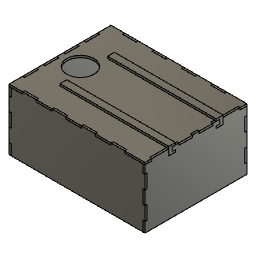
prototype v2 (Autodesk Fusion 360 design; units mm, degrees)
Autodesk Fusion 360 part; units mm, degrees
note: some values were not read from the file. Set by a fixed rule: which sketch regions a step uses.
sketch "Sketch1" plane through (0, 0, 0) normal (0, 1, 0) x (1, 0, 0)
  line L0 (0, 0) -> (200, 0)
  line L1 (200, 0) -> (200, -150)
  line L2 (200, -150) -> (0, -150)
  line L3 (0, -150) -> (0, 0)
  line L4 (0, -20) -> (3, -20)
  line L5 (3, -20) -> (3, -40)
  line L6 (3, -40) -> (0, -40)
  line L7 (0, -40) -> (0, -20)
  line L8 (3, -70) -> (0, -70)
  line L9 (3, -50) -> (3, -70)
  line L10 (0, -50) -> (3, -50)
  line L11 (3, -100) -> (0, -100)
  line L12 (3, -80) -> (3, -100)
  line L13 (0, -80) -> (3, -80)
  line L14 (3, -130) -> (0, -130)
  line L15 (3, -110) -> (3, -130)
  line L16 (0, -110) -> (3, -110)
  line L17 (170, 0) -> (150, 0)
  line L18 (150, 0) -> (150, -3)
  line L19 (150, -3) -> (170, -3)
  line L20 (170, -3) -> (170, 0)
  line L21 (170, -150) -> (150, -150)
  line L22 (150, -150) -> (150, -147)
  line L23 (150, -147) -> (170, -147)
  line L24 (170, -147) -> (170, -150)
  line L25 (-40, -147) -> (-40, -150)
  line L26 (200, -40) -> (200, -35)
  line L27 (200, -110) -> (40, -110)
  line L28 (40, -110) -> (40, -115)
  line L29 (40, -115) -> (200, -115)
  line L30 (200, -115) -> (200, -110)
  line L31 (200, -120) -> (200, -140)
  line L32 (200, -10.0504) -> (197, -10.0504)
  line L33 (197, -10.0504) -> (197, -30.0504)
  line L34 (197, -30.0504) -> (200, -30.0504)
  line L35 (200, -30.0504) -> (200, -10.0504)
  line L36 (200, -50) -> (197, -50)
  line L37 (197, -50) -> (197, -70)
  line L38 (197, -70) -> (200, -70)
  line L39 (200, -70) -> (200, -50)
  line L40 (200, -80) -> (197, -80)
  line L41 (197, -80) -> (197, -100)
  line L42 (197, -100) -> (200, -100)
  line L43 (30, 0) -> (30, -150) construction
  line L44 (0, -75) -> (30, -75) construction
  circle A0 centre (30, -75) radius 20
  line L45 (46.6667, -115) -> (53.3333, -110) construction
  line L46 (200, -35) -> (40, -35)
  line L47 (40, -35) -> (40, -40)
  line L48 (40, -40) -> (200, -40)
  line L49 (200, -40) -> (200, -35)
  line L50 (106.6667, -3) -> (126.6667, -3)
  line L51 (106.6667, 0) -> (106.6667, -3)
  line L52 (126.6667, -3) -> (126.6667, 0)
  line L53 (63.3333, -3) -> (83.3333, -3)
  line L54 (63.3333, 0) -> (63.3333, -3)
  line L55 (83.3333, -3) -> (83.3333, 0)
  line L56 (20, -3) -> (40, -3)
  line L57 (20, 0) -> (20, -3)
  line L58 (40, -3) -> (40, 0)
  line L59 (106.6667, -147) -> (126.6667, -147)
  line L60 (126.6667, -147) -> (126.6667, -150)
  line L61 (106.6667, -150) -> (106.6667, -147)
  line L62 (63.3333, -147) -> (83.3333, -147)
  line L63 (83.3333, -147) -> (83.3333, -150)
  line L64 (63.3333, -150) -> (63.3333, -147)
  line L65 (20, -147) -> (40, -147)
  line L66 (40, -147) -> (40, -150)
  line L67 (20, -150) -> (20, -147)
  line L68 (200, -120) -> (197, -120)
  line L69 (197, -120) -> (197, -140)
  line L70 (197, -140) -> (200, -140)
  line L71 (200, -140) -> (200, -120)
  line L72 (197, -150) -> (197, 0)
  point P0 (0, -20)
  point P1 (170, 0)
  point P2 (170, -150)
  point P3 (200, -35)
  point P4 (200, -110)
  point P5 (30, 0)
  point P6 (197, -150)
  dimension "d1" = 200
  dimension "d2" = 150
  dimension "d10" = 20
  dimension "d11" = 3
  dimension "d12" = 20
  dimension "d15" = 0
  dimension "d16" = -90
  dimension "d17" = 30
  dimension "d18" = 20
  dimension "d19" = 3
  dimension "d24" = 30
  dimension "d25" = 20
  dimension "d31" = 35
  dimension "d37" = 70
  dimension "d39" = 5
  dimension "d44" = 3
  dimension "d48" = 0
  dimension "d49" = -30
  dimension "d155" = 30
  dimension "d157" = 40
  dimension "d158" = 160
  dimension "d162" = -130
  dimension "d163" = 0
  dimension "d166" = -130
  dimension "d167" = 0
  constraint horizontal L0
  constraint vertical L1
  constraint horizontal L2
  constraint vertical L3
  constraint coincident L0.start L3.end
  constraint coincident L3 P0
  constraint horizontal L4
  constraint vertical L5
  constraint horizontal L6
  constraint vertical L7
  constraint coincident P0 L4.start
  constraint coincident L0 P1
  constraint horizontal L17
  constraint vertical L18
  constraint horizontal L19
  constraint vertical L20
  constraint coincident P1 L17.start
  constraint coincident L2 P2
  constraint horizontal L21
  constraint vertical L22
  constraint horizontal L23
  constraint vertical L24
  constraint coincident P2 L21.start
  constraint coincident L1 P3
  constraint vertical L26
  constraint coincident P3 L26.end
  constraint coincident L1 P4
  constraint horizontal L27
  constraint vertical L28
  constraint horizontal L29
  constraint vertical L30
  constraint coincident P4 L27.start
  constraint vertical L31
  constraint coincident L1 L31.end
  constraint horizontal L32
  constraint vertical L33
  constraint horizontal L34
  constraint vertical L35
  constraint coincident L1 L32.start
  constraint horizontal L36
  constraint vertical L37
  constraint horizontal L38
  constraint vertical L39
  constraint coincident L1 L36.start
  constraint coincident L0 P5
  constraint coincident P5 L43.start
  constraint coincident L2 L43.end
  constraint perpendicular L2 L43
  constraint midpoint L3 L44.start
  constraint midpoint L43 L44.end
  constraint coincident L44.end A0.centre
  constraint coincident L27 L45.end
  constraint coincident L29 L45.start
  constraint horizontal L46
  constraint vertical L47
  constraint horizontal L48
  constraint vertical L49
  constraint horizontal L68
  constraint vertical L69
  constraint horizontal L70
  constraint vertical L71
  constraint coincident L2 P6
  constraint coincident P6 L72.start
  measures "d1" distance of L0.start L0.end
  measures "d2" distance of L0.start L2.end
  measures "d10" distance of L0.start L4.start
  measures "d11" distance of P0 L4.end
  measures "d12" distance of P0 L6.end
  measures "d17" distance of L1 P1
  measures "d18" distance of P1 L17.end
  measures "d19" distance of P1 L19.end
  measures "d24" distance of L1.end P2
  measures "d25" distance of P2 L21.end
  measures "d31" distance of L0.end P3
  measures "d37" distance of L26.start P4
  measures "d39" distance of P4 L29.end
  measures "d44" distance of L36.start L36.end
  measures "d155" distance of L0.start P5
  measures "d157" diameter of A0
  measures "d158" distance of P3 L46.end
extrude "Extrude1" add sketch "Sketch1" against normal blind 3 contours L0 L2 L3 L4 L5 L6 L8 L9 L10 L11 L12 L13 L14 L15 L16 L18 L19 L20 L22 L23 L24 L27 L28 L29 L33 L37 L41 L46 L47 L48 L50 L51 L52 L53 L54 L55 L56 L57 L58 L59 L60 L61 L62 L63 L64 L65 L66 L67 L69 L72 | L0 L1 L32 L72 | L1 L36 L37 L38 L39 L72 | L1 L40 L41 L42 L72 | L1 L2 L70 L72 makes body 1
sketch "Sketch2" plane through (0, 0, 150) normal (0, 0, 1) x (1, 0, 0)
  line L0 (200, 0) -> (200, -90)
  line L1 (200, -90) -> (0, -90)
  line L2 (0, -90) -> (0, 0)
  line L3 (0, -3) -> (0, 0)
  line L4 (200, -3) -> (200, 0)
  line L5 (0, -35) -> (0, -15)
  line L6 (0, -15) -> (3, -15)
  line L7 (3, -15) -> (3, -35)
  line L8 (3, -35) -> (0, -35)
  line L9 (0, -35) -> (0, -15)
  line L10 (0, -55) -> (3, -55)
  line L11 (3, -55) -> (3, -75)
  line L12 (3, -75) -> (0, -75)
  line L13 (3, -35) -> (3, -55)
  line L14 (3, -75) -> (3, -90)
  line L15 (200, -15) -> (197, -15)
  line L16 (197, -15) -> (197, -35)
  line L17 (197, -35) -> (200, -35)
  line L18 (200, -35) -> (200, -15)
  line L19 (200, -55) -> (197, -55)
  line L20 (197, -55) -> (197, -75)
  line L21 (197, -75) -> (200, -75)
  line L22 (0, 0) -> (200, 0)
  line L23 (3, -15) -> (3, 0)
  line L24 (170, 0) -> (150, 0)
  line L25 (150, 0) -> (150, -3)
  line L26 (150, -3) -> (170, -3)
  line L27 (170, -3) -> (170, 0)
  line L28 (106.6667, -3) -> (126.6667, -3)
  line L29 (106.6667, 0) -> (106.6667, -3)
  line L30 (126.6667, -3) -> (126.6667, 0)
  line L31 (63.3333, -3) -> (83.3333, -3)
  line L32 (63.3333, 0) -> (63.3333, -3)
  line L33 (83.3333, -3) -> (83.3333, 0)
  line L34 (20, -3) -> (40, -3)
  line L35 (20, 0) -> (20, -3)
  line L36 (40, -3) -> (40, 0)
  line L37 (200, -3) -> (0, -3)
  line L38 (197, -3) -> (197, -90)
  point P0 (0, -15)
  point P1 (0, -55)
  point P2 (200, -15)
  point P3 (0, -3)
  point P4 (200, -3)
  point P5 (170, 0)
  point P6 (197, -3)
  dimension "d61" = 200
  dimension "d62" = 90
  dimension "d98" = 15
  dimension "d105" = 0
  dimension "d106" = -40
  dimension "d116" = 20
  dimension "d119" = 0
  dimension "d120" = -40
  dimension "d180" = -130
  dimension "d181" = 0
  constraint vertical L0
  constraint vertical L2
  constraint coincident L2.end L3.end
  constraint vertical L3
  constraint vertical L4
  constraint coincident L2 P0
  constraint vertical L5
  constraint coincident P0 L5.end
  constraint horizontal L6
  constraint vertical L7
  constraint horizontal L8
  constraint vertical L9
  constraint coincident L2 P1
  constraint coincident L1 L14.end
  constraint coincident L0 P2
  constraint horizontal L15
  constraint vertical L16
  constraint horizontal L17
  constraint vertical L18
  constraint coincident P2 L15.start
  constraint perpendicular L0 L22
  constraint coincident L22 L23.end
  constraint perpendicular L22 L23
  constraint horizontal L24
  constraint vertical L25
  constraint horizontal L26
  constraint vertical L27
  constraint coincident P5 L24.start
  constraint coincident P4 L4.start
  constraint perpendicular L0 L37
  constraint coincident L37 P6
  constraint coincident P6 L38.start
  constraint coincident L1 L38.end
  constraint perpendicular L1 L38
  measures "d61" distance of L2.end L0.start
  measures "d62" distance of L2.end L1.end
  measures "d98" distance of L2.end L5.end
  measures "d116" distance of P2 L17.end
extrude "Extrude4" add sketch "Sketch2" against normal blind 3 separate body contours L22 L24 L25 L26 L27 L37 | L0 L15 L16 L17 L18 L38 | L1 L7 L11 L13 L14 L16 L20 L23 L26 L28 L31 L34 L37 L38 | L22 L28 L29 L30 L37 | L0 L19 L20 L21 L38 | L22 L31 L32 L33 L37 | L22 L34 L35 L36 L37 | L2 L10 L11 L12 | L2 L5 L6 L7 L8 L9 makes body 2
sketch "Sketch3" plane through (0, 0, 0) normal (0, 0, -1) x (-1, 0, 0)
  line L0 (-200, 0) -> (-200, -90)
  line L1 (-200, -90) -> (0, -90)
  line L2 (0, -90) -> (0, 0)
  line L3 (-200, -3) -> (-200, 0)
  line L4 (0, -3) -> (0, 0)
  line L5 (-3, -15) -> (-3, 0)
  line L6 (-3, -15) -> (-3, -90)
  line L7 (-3, -15) -> (0, -15)
  line L8 (-3, -35) -> (0, -35)
  line L9 (-3, -55) -> (0, -55)
  line L10 (0, -75) -> (-3, -75)
  line L11 (-200, -15) -> (-197, -15)
  line L12 (-197, -15) -> (-197, -35)
  line L13 (-197, -35) -> (-200, -35)
  line L14 (-200, -35) -> (-200, -15)
  line L15 (-170, 0) -> (-150, 0)
  line L16 (-150, 0) -> (-150, -3)
  line L17 (-150, -3) -> (-170, -3)
  line L18 (-170, -3) -> (-170, 0)
  line L19 (-126.6667, -3) -> (-126.6667, 0)
  line L20 (-106.6667, -3) -> (-126.6667, -3)
  line L21 (-106.6667, 0) -> (-106.6667, -3)
  line L22 (-83.3333, -3) -> (-83.3333, 0)
  line L23 (-63.3333, -3) -> (-83.3333, -3)
  line L24 (-63.3333, 0) -> (-63.3333, -3)
  line L25 (-40, -3) -> (-40, 0)
  line L26 (-20, -3) -> (-40, -3)
  line L27 (-20, 0) -> (-20, -3)
  line L28 (-200, -90) -> (-3, -90)
  line L29 (-200, 0) -> (0, 0)
  line L30 (0, -3) -> (-200, -3)
  line L31 (-200, -55) -> (-197, -55)
  line L32 (-197, -55) -> (-197, -75)
  line L33 (-197, -75) -> (-200, -75)
  line L34 (-200, -75) -> (-200, -55)
  line L35 (-197, -90) -> (-197, 0)
  point P0 (-3, -35)
  point P1 (-3, -55)
  point P2 (-3, -75)
  point P3 (-200, -15)
  point P4 (0, -3)
  point P5 (-170, 0)
  point P6 (-150, -3)
  point P7 (-3, -15)
  point P8 (0, -15)
  point P9 (-200, -55)
  point P10 (-197, -90)
  dimension "d65" = 200
  dimension "d66" = 90
  dimension "d108" = 3
  dimension "d172" = 130
  dimension "d173" = 0
  constraint vertical L0
  constraint coincident L2.end L4.end
  constraint coincident L2 P8
  constraint coincident P0 L8.start
  constraint coincident L2 L8.end
  constraint coincident P1 L9.start
  constraint coincident L2 L9.end
  constraint coincident L2 L10.start
  constraint coincident P2 L10.end
  constraint perpendicular L6 L10
  constraint coincident L0 P3
  constraint horizontal L11
  constraint vertical L12
  constraint horizontal L13
  constraint vertical L14
  constraint coincident P3 L11.start
  constraint horizontal L15
  constraint vertical L16
  constraint horizontal L17
  constraint vertical L18
  constraint coincident P6 L16.end
  constraint coincident P5 L15.start
  constraint perpendicular L2 L29
  constraint perpendicular L3 L30
  constraint horizontal L31
  constraint vertical L32
  constraint horizontal L33
  constraint vertical L34
  constraint coincident P9 L31.start
  constraint coincident P10 L35.start
  constraint coincident L29 L35.end
  measures "d65" distance of L2.end L0.start
  measures "d66" distance of L2.end L1.end
  measures "d108" distance of P3 L11.end
extrude "Extrude12" add sketch "Sketch3" against normal blind 3 separate body contours L0 L11 L12 L13 L14 L35 | L1 L5 L6 L12 L17 L20 L23 L26 L28 L30 L32 L35 | L15 L16 L17 L18 L29 L30 | L0 L31 L32 L33 L34 L35 | L19 L20 L21 L29 L30 | L22 L23 L24 L29 L30 | L25 L26 L27 L29 L30 | L2 L6 L9 L10 | L2 L6 L7 L8 makes body 3
sketch "Sketch4" plane through (200, 0, 0) normal (1, 0, 0) x (0, 0, -1)
  line L0 (-140, 0) -> (-150, 0)
  line L1 (-150, 0) -> (-150, -3)
  line L2 (-150, -3) -> (-140, -3)
  line L3 (0, 0) -> (-150, 0)
  line L4 (-150, 0) -> (-150, -90)
  line L5 (-150, -90) -> (0, -90)
  line L6 (0, -90) -> (0, 0)
  line L7 (-10.0504, -3) -> (0, -3)
  line L8 (0, -3) -> (0, 0)
  line L9 (0, 0) -> (-10.0504, 0)
  line L10 (-10.0504, 0) -> (-10.0504, -3)
  line L11 (-30.0504, -3) -> (-35, -3)
  line L12 (-35, -3) -> (-35, 0)
  line L13 (-35, 0) -> (-30.0504, 0)
  line L14 (-30.0504, 0) -> (-30.0504, -3)
  line L15 (-40, -3) -> (-50, -3)
  line L16 (-50, -3) -> (-50, 0)
  line L17 (-50, 0) -> (-40, 0)
  line L18 (-40, 0) -> (-40, -3)
  line L19 (-70, -3) -> (-80, -3)
  line L20 (-80, -3) -> (-80, 0)
  line L21 (-80, 0) -> (-70, 0)
  line L22 (-70, 0) -> (-70, -3)
  line L23 (-100, -3) -> (-110, -3)
  line L24 (-110, -3) -> (-110, 0)
  line L25 (-110, 0) -> (-100, 0)
  line L26 (-100, 0) -> (-100, -3)
  line L27 (-115, -3) -> (-120, -3)
  line L28 (-120, -3) -> (-120, 0)
  line L29 (-120, 0) -> (-115, 0)
  line L30 (-115, 0) -> (-115, -3)
  line L31 (-140, -3) -> (-150, -3)
  line L32 (-150, -3) -> (-150, 0)
  line L33 (-150, 0) -> (-140, 0)
  line L34 (-140, 0) -> (-140, -3)
  line L35 (-115, -3) -> (-110, -3)
  line L36 (-40, -3) -> (-35, -3)
  line L37 (-115, -3) -> (-110, -3)
  line L38 (-35, -3) -> (-45, -3)
  line L39 (-150, -15) -> (-147, -15)
  line L40 (-147, -15) -> (-147, -35)
  line L41 (-147, -35) -> (-150, -35)
  line L42 (-150, -35) -> (-150, -15)
  line L43 (-150, -55) -> (-147, -55)
  line L44 (-147, -55) -> (-147, -75)
  line L45 (-147, -75) -> (-150, -75)
  line L46 (-147, -15, 0) -> (-147, -90, -3)
  line L47 (-147, -15) -> (-147, 0)
  line L48 (0, -15) -> (-3, -15)
  line L49 (-3, -15) -> (-3, -35)
  line L50 (-3, -35) -> (0, -35)
  line L51 (0, -35) -> (0, -15)
  line L52 (0, -55) -> (-3, -55)
  line L53 (-3, -55) -> (-3, -75)
  line L54 (-3, -75) -> (0, -75)
  line L55 (-3.0756, 0) -> (-3.0756, -90)
  line L56 (-115, -3) -> (-105, -3)
  line L57 (-105, -9) -> (-115, -9)
  line L58 (-115, -9) -> (-115, -3)
  line L59 (-35, -3) -> (-45, -3)
  line L60 (-45, -9) -> (-35, -9)
  line L61 (-35, -9) -> (-35, -3)
  line L62 (-110, -3) -> (-110, -6)
  line L63 (-110, -6) -> (-105, -6)
  line L64 (-105, -6) -> (-105, -9)
  line L65 (-40, -3) -> (-40, -6)
  line L66 (-40, -6) -> (-45, -6)
  line L67 (-45, -6) -> (-45, -9)
  line L68 (-115, 0) -> (-104.994, 0)
  line L69 (-104.994, 0) -> (-104.994, 3)
  line L70 (-104.994, 3) -> (-115, 3)
  line L71 (-115, 3) -> (-115, 0)
  line L72 (-35, 0) -> (-45, 0)
  line L73 (-45, 0) -> (-45, 3)
  line L74 (-45, 3) -> (-35, 3)
  line L75 (-35, 3) -> (-35, 0)
  line L76 (-140, -3) -> (-140, 0)
  line L77 (-150, -3) -> (0, -3)
  point P0 (-70, -3)
  point P1 (-30.0504, -3)
  point P2 (-10.0504, -3)
  point P3 (-150, -15)
  point P4 (0, -15)
  point P5 (-115, -3)
  point P6 (-115, 0)
  point P7 (-147, -90)
  point P8 (-30.0504, -3)
  point P9 (-30.0504, 0)
  point P10 (-150, -3)
  point P11 (-140, -3)
  point P12 (-120, -3)
  point P13 (-35, -3)
  point P14 (-35, 0)
  point P15 (-120, 0)
  point P16 (-115, -3)
  point P17 (-110, -3)
  point P18 (-100, -3)
  point P19 (-80, -3)
  point P20 (-50, -3)
  point P21 (-50, -3)
  point P22 (-70, -3)
  point P23 (-50, 0)
  point P24 (-80, 0)
  point P25 (-110, 0)
  point P26 (-110, 0)
  point P27 (-150, -15)
  point P28 (-147, -90)
  dimension "d69" = 150
  dimension "d70" = 90
  dimension "d79" = 10
  dimension "d122" = 3
  dimension "d123" = 20
  dimension "d126" = 0
  dimension "d127" = -40
  dimension "d129" = 3
  dimension "d130" = 20
  dimension "d133" = 0
  dimension "d134" = -40
  dimension "d143" = 10
  dimension "d144" = 6
  dimension "d145" = 10
  dimension "d146" = 6
  dimension "d147" = 3
  dimension "d153" = 3
  dimension "d154" = 3
  dimension "d185" = 150
  constraint horizontal L3
  constraint vertical L4
  constraint horizontal L5
  constraint vertical L6
  constraint coincident L3.start L6.end
  constraint horizontal L7
  constraint vertical L8
  constraint horizontal L9
  constraint vertical L10
  constraint coincident P2 L7.start
  constraint horizontal L11
  constraint vertical L12
  constraint horizontal L13
  constraint vertical L14
  constraint coincident P8 P1
  constraint horizontal L15
  constraint vertical L16
  constraint horizontal L17
  constraint vertical L18
  constraint horizontal L19
  constraint vertical L20
  constraint horizontal L21
  constraint vertical L22
  constraint coincident P22 P0
  constraint horizontal L23
  constraint vertical L24
  constraint horizontal L25
  constraint vertical L26
  constraint horizontal L27
  constraint vertical L28
  constraint horizontal L29
  constraint vertical L30
  constraint horizontal L31
  constraint vertical L32
  constraint horizontal L33
  constraint vertical L34
  constraint coincident L0.end L1.start
  constraint coincident P17 L23.end
  constraint horizontal L37
  constraint horizontal L38
  constraint horizontal L39
  constraint vertical L40
  constraint horizontal L41
  constraint vertical L42
  constraint coincident L3 L47.end
  constraint coincident L6 P4
  constraint horizontal L48
  constraint vertical L49
  constraint horizontal L50
  constraint vertical L51
  constraint coincident P4 L48.start
  constraint coincident L3 L55.start
  constraint coincident L5 L55.end
  constraint perpendicular L5 L55
  constraint horizontal L56
  constraint horizontal L57
  constraint vertical L58
  constraint horizontal L59
  constraint horizontal L60
  constraint vertical L61
  constraint perpendicular L56 L62
  constraint perpendicular L62 L63
  constraint perpendicular L38 L65
  constraint perpendicular L65 L66
  constraint horizontal L68
  constraint vertical L69
  constraint horizontal L70
  constraint vertical L71
  constraint horizontal L72
  constraint vertical L73
  constraint horizontal L74
  constraint vertical L75
  constraint perpendicular L4 L77
  measures "d69" distance of L3.start L0.end
  measures "d70" distance of L3.start L5.end
  measures "d79" distance of P13 L38.end
  measures "d122" distance of P27 L39.end
  measures "d123" distance of P27 L41.end
  measures "d129" distance of P4 L48.end
  measures "d130" distance of P4 L50.end
  measures "d143" distance of P16 L56.end
  measures "d144" distance of P16 L57.end
  measures "d145" distance of P13 L38.end
  measures "d146" distance of P13 L60.end
  measures "d147" distance of P17 L62.end
  measures "d153" distance of P6 L70.end
  measures "d154" distance of P14 L74.end
  measures "d185" distance of P10 L7.end
extrude "Extrude6" add sketch "Sketch4" against normal blind 3 separate body contours L3 L28 L34 L76 L77 | L3 L27 L28 L29 L30 L77 | L2 L4 L5 L7 L11 L15 L19 L23 L27 L31 L38 L40 L41 L43 L44 L45 L47 L55 L56 L57 L58 L59 L60 L61 L62 L63 L64 L65 L66 L67 L77 | L2 L4 L31 L39 L47 L77 | L3 L23 L24 L25 L26 L56 L68 L77 | L3 L19 L20 L21 L22 L77 | L3 L15 L16 L17 L18 L38 L59 L72 L77 | L5 L6 L7 L48 L49 L50 L52 L53 L54 L55 L77 | L3 L10 L14 L77 | L3 L11 L12 L13 L14 L77 makes body 4
sketch "Sketch5" plane through (0, 0, 0) normal (-1, 0, 0) x (0, 0, 1)
  line L0 (50, 0) -> (40, 0)
  line L1 (40, 0) -> (40, -3)
  line L2 (40, -3) -> (50, -3)
  line L3 (50, -3) -> (50, 0)
  line L4 (0, 0) -> (150, 0)
  line L5 (150, 0) -> (150, -90)
  line L6 (150, -90) -> (0, -90)
  line L7 (0, -90) -> (0, 0)
  line L8 (130, -3) -> (150, -3)
  line L9 (150, -3) -> (150, 0)
  line L10 (150, 0) -> (130, 0)
  line L11 (130, 0) -> (130, -3)
  line L12 (110, -3) -> (100, -3)
  line L13 (100, -3) -> (100, 0)
  line L14 (100, 0) -> (110, 0)
  line L15 (110, 0) -> (110, -3)
  line L16 (80, -3) -> (70, -3)
  line L17 (70, -3) -> (70, 0)
  line L18 (70, 0) -> (80, 0)
  line L19 (80, 0) -> (80, -3)
  line L20 (50, -3) -> (40, -3)
  line L21 (40, -3) -> (40, 0)
  line L22 (40, 0) -> (50, 0)
  line L23 (50, 0) -> (50, -3)
  line L24 (20, -3) -> (0, -3)
  line L25 (0, -3) -> (0, 0)
  line L26 (0, 0) -> (20, 0)
  line L27 (20, 0) -> (20, -3)
  line L28 (150, -15) -> (147, -15)
  line L29 (147, -15) -> (147, -35)
  line L30 (147, -35) -> (150, -35)
  line L31 (150, -35) -> (150, -15)
  line L32 (150, -55) -> (147, -55)
  line L33 (147, -55) -> (147, -75)
  line L34 (147, -75) -> (150, -75)
  line L35 (0, -15) -> (3, -15)
  line L36 (3, -15) -> (3, -35)
  line L37 (3, -35) -> (0, -35)
  line L38 (0, -35) -> (0, -15)
  line L39 (0, -55) -> (3, -55)
  line L40 (3, -55) -> (3, -75)
  line L41 (3, -75) -> (0, -75)
  line L42 (3, -15) -> (3, -35)
  line L43 (3, -55) -> (3, -75)
  circle A0 centre (125, -25) radius 7.5
  point P0 (20, -3)
  point P1 (40, -3)
  point P2 (50, -3)
  point P3 (70, -3)
  point P4 (80, -3)
  point P5 (100, -3)
  point P6 (110, -3)
  point P7 (130, -3)
  point P8 (100, 0)
  point P9 (70, 0)
  point P10 (150, -15)
  point P11 (0, -15)
  point P12 (125, -25)
  dimension "d73" = 150
  dimension "d74" = 90
  dimension "d85" = 15
  dimension "d86" = 3
  dimension "d90" = 0
  dimension "d91" = -40
  dimension "d96" = 0
  dimension "d97" = -40
  dimension "d141" = 15
  constraint horizontal L4
  constraint vertical L5
  constraint horizontal L6
  constraint vertical L7
  constraint coincident L4.start L7.end
  constraint horizontal L8
  constraint vertical L9
  constraint horizontal L10
  constraint vertical L11
  constraint coincident P7 L8.start
  constraint horizontal L12
  constraint vertical L13
  constraint horizontal L14
  constraint vertical L15
  constraint coincident P8 L13.end
  constraint coincident P6 L12.start
  constraint horizontal L16
  constraint vertical L17
  constraint horizontal L18
  constraint vertical L19
  constraint coincident P9 L17.end
  constraint coincident P4 L16.start
  constraint horizontal L20
  constraint vertical L21
  constraint horizontal L22
  constraint vertical L23
  constraint coincident L0.end L1.start
  constraint coincident P2 L2.end
  constraint horizontal L24
  constraint vertical L25
  constraint horizontal L26
  constraint vertical L27
  constraint coincident P0 L24.start
  constraint coincident L5 P10
  constraint horizontal L28
  constraint vertical L29
  constraint horizontal L30
  constraint vertical L31
  constraint coincident P10 L28.start
  constraint coincident L7 P11
  constraint horizontal L35
  constraint vertical L36
  constraint horizontal L37
  constraint vertical L38
  constraint coincident P11 L35.start
  constraint coincident P12 A0.centre
  measures "d73" distance of L4.start L4.end
  measures "d74" distance of L4.start L6.end
  measures "d85" distance of L4.end P10
  measures "d86" distance of P10 L28.end
  measures "d141" diameter of A0
extrude "Extrude7" add sketch "Sketch5" against normal blind 3 separate body contours L1 L2 L3 L4 L5 L6 L7 L8 L11 L12 L13 L15 L16 L17 L19 L20 L21 L23 L24 L27 L28 L29 L30 L32 L33 L34 L35 L36 L37 L39 L40 L41 L42 L43 makes body 5
extrude "Extrude8" cut sketch "Sketch4" against normal blind 3 contours L3 L24 L30 L35 L37 L56 L68 L77 | L3 L12 L18 L36 L38 L59 L72 L77
extrude "Extrude9" add sketch "Sketch4" along normal blind 160 separate body contours L3 L25 L68 L69 L70 L71 | L3 L24 L30 L35 L37 L56 L68 L77 | L35 L37 L56 L57 L58 L62 L63 L64 L77 | L3 L17 L72 L73 L74 L75 | L3 L12 L18 L36 L38 L59 L72 L77 | L36 L38 L59 L60 L61 L65 L66 L67 L77 makes body 6 at (253.3333, -1, 115) makes body 7 at (253.3333, -5, 35)
move_body "Move20" bodies 6 7 to x (1, 0, 0) y (0, 1, 0) z (0, 0, 1) at (-160, 0, 0)
move_body "Move16" [suppressed]
move_body "Move17" [suppressed]
move_body "Move18" [suppressed]
move_body "Move19" [suppressed]
equation "d1 = length"
equation "d2 = width"
equation "length = 200 mm" comment "length of entire body"
equation "width = 150 mm" comment "entire body width"
equation "bRadius = 40 mm" comment "bulb holder radius"
equation "girth = 3 mm" comment "material thickness"
equation "fit = 20 mm" comment "length of fit cuts"
equation "d11 = girth"
equation "d12 = fit"
equation "d18 = fit"
equation "d19 = girth"
equation "d25 = fit"
equation "holderL = 160 mm" comment "PCB holder length"
equation "holderW = 5 mm" comment "PCB holder width"
equation "pcbW = 70 mm" comment "PCB width"
equation "d37 = pcbW"
equation "d39 = holderW"
equation "d44 = girth"
equation "d50 = -girth"
equation "bLength = 40 mm" comment "bulb holder length"
equation "bottomClearence = 50 mm" comment "from bulb holder to floor"
equation "d61 = length"
equation "d62 = bottomClearence + bLength"
equation "d63 = -girth"
equation "d65 = length"
equation "d66 = bottomClearence + bLength"
equation "d69 = width"
equation "d70 = bottomClearence + bLength"
equation "d71 = -girth"
equation "d73 = width"
equation "d74 = bottomClearence + bLength"
equation "d75 = -girth"
equation "d79 = holderW + 5 mm"
equation "d81 = -girth"
equation "d83 = holderL"
equation "d86 = girth"
equation "d108 = girth"
equation "d116 = fit"
equation "d122 = girth"
equation "d123 = fit"
equation "d129 = girth"
equation "d130 = fit"
equation "wireH = 15 mm" comment "wire hole"
equation "entryT = 70 mm" comment "wire entry top"
equation "entryS = 50 mm" comment "wire entry side"
equation "d141 = wireH"
equation "pcbC = 3 mm" comment "PCB cleareance"
equation "d144 = pcbC + 3 mm"
equation "d146 = pcbC + 3 mm"
equation "d147 = pcbC"
equation "d153 = girth"
equation "d154 = girth"
equation "d155 = centerOffset"
equation "centerOffset = bRadius * 0.5 + 10 mm" comment "from edge to circle center"
equation "d157 = bRadius"
equation "d158 = holderL"
equation "d174 = -girth"
equation "d185 = width"
named bodies: "top", "left", "leftHolder", "rightHolder", "front", "back", "right"
